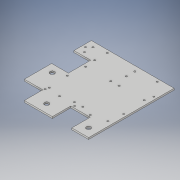
# Autodesk Inventor part: КВ33.044.002 - Дно платы
Saved by Autodesk Inventor 2019 (Build 230136000, 136)
## iProperties
Created: 2019-10-30
Part Number: КВ33.044.002 - Дно платы
Material: Типовые
Document SubType Name: Modeling
Designer: Петров Иван
Density: 1 g/cm^3
Appearance: По умолчанию
Mass: 56.5933 g
Surface Area: 408.613 cm^2
Volume: 56.5933 cm^3
Author: Петров Иван
Autodesk Inventor part; units mm, degrees
ref_plane "YZ Plane" through (0, 0, 0) normal (1, 0, 0) x (0, 1, 0)
ref_plane "XZ Plane" through (0, 0, 0) normal (0, 1, 0) x (-1, 0, 0)
ref_plane "XY Plane" through (0, 0, 0) normal (0, 0, 1) x (1, 0, 0)
sketch "Эскиз1" plane through (0, 0, 0) normal (0, 1, 0) x (-1, 0, 0)
  line L0 (-25, 35) -> (25, 35)
  line L1 (25, 35) -> (25, -35)
  line L2 (25, -35) -> (-25, -35)
  line L3 (-25, -35) -> (-25, 35)
  line L4 (-22.5, 32.5) -> (22.5, 32.5)
  line L5 (22.5, 31.5) -> (22.5, -31)
  line L6 (22.5, -32.5) -> (-22.5, -32.5)
  circle A0 centre (22.5, 32.5) radius 1.5
  circle A1 centre (22.5, -32.5) radius 1.5
  circle A2 centre (-22.5, -32.5) radius 1.5
  circle A3 centre (-22.5, 32.5) radius 1.5
  line L7 (-25, 35) -> (-23.7767, 33.2874) construction
  line L8 (-22.5, -31) -> (-22.5, 31)
  line L9 (23.7767, -33.2874) -> (25, -35) construction
  line L10 (25, -30.9585) -> (25, 35)
  line L11 (25, 35) -> (-25, 35)
  line L12 (25, 35) -> (25, -35)
  point P0 (0, 0)
  dimension "d6" = 3
  dimension "d0" = 50
  dimension "d2" = 45
  dimension "d4" = 3
  dimension "d5" = 3
  dimension "d7" = 3
  constraints: 26 end point, 4 coincident, 4 parallel, 4 point on circle, 3 centre point, 3 horizontal, 2 perpendicular, 2 point on line, 1 vertical alignment, 2 other
  measures "d0" distance of L1.end L2.end
  measures "d2" distance of L6.start L6.end
  measures "d4" diameter of A0
  measures "d5" diameter of A1
  measures "d7" diameter of A3
extrude "Выдавливание1" add sketch "Эскиз1" along normal blind 3 contours L0 L1 L2 L3 | L4 A0 L5 A1 L6 A2 L8 A3
sketch "Эскиз2" plane through (0, 3, 0) normal (0, 1, 0) x (1, 0, 0)
  line L0 (-25, -35) -> (25, -35) projected
  line L1 (-25, -35) -> (-28, -35)
  line L2 (-28, -35) -> (-28, 35)
  line L3 (-28, 35) -> (-25, 35)
  line L4 (-25, 35) -> (-25, -35)
  line L5 (-28, -35) -> (-58, -35)
  line L6 (-58, -35) -> (-58, 35)
  line L7 (-58, 35) -> (-28, 35)
  line L8 (-28, 35) -> (-28, -35)
  line L9 (-25, -35) -> (25, -35)
  line L10 (25, -35) -> (25, -38)
  line L11 (25, -38) -> (-25, -38)
  line L12 (-25, -38) -> (-25, -35)
  line L13 (-25, -38) -> (25, -38)
  line L14 (25, -38) -> (25, -68)
  line L15 (25, -68) -> (-25, -68)
  line L16 (-25, -68) -> (-25, -38)
  line L17 (-25, -68) -> (0, -68)
  line L18 (0, -53) -> (-25, -53)
  line L19 (-25, -53) -> (-25, -68)
  circle A0 centre (0, -53) radius 4
  line L20 (-58, 0) -> (-43, 0)
  circle A1 centre (-43, 0) radius 4
  point P0 (0, 0)
  dimension "d18" = 3
  dimension "d19" = 70
  dimension "d20" = 30
  dimension "d21" = 70
  dimension "d22" = 50
  dimension "d23" = 3
  dimension "d24" = 50
  dimension "d25" = 30
  dimension "d26" = 25
  dimension "d27" = 15
  dimension "d28" = 8
  dimension "d29" = 15
  dimension "d30" = 8
  constraints: 40 end point, 9 parallel, 6 horizontal, 4 perpendicular, 2 centre point, 2 coincident, 1 midpoint
  measures "d18" distance of L2.end L3.end
  measures "d19" distance of L1.end L2.end
  measures "d20" distance of L6.end L7.end
  measures "d21" distance of L5.end L6.end
  measures "d22" distance of L10.end L11.end
  measures "d23" distance of L9.end L10.end
  measures "d24" distance of L14.end L15.end
  measures "d25" distance of L13.end L14.end
  measures "d26" distance of L18.end L18.start
  measures "d27" distance of L18.start L17.end
  measures "d28" diameter of A0
  measures "d29" distance of L20.start L20.end
  measures "d30" diameter of A1
extrude "Выдавливание2" add sketch "Эскиз2" against normal blind 3
sketch "Эскиз3" plane through (0, 3, 0) normal (0, 1, 0) x (1, 0, 0)
  line L0 (-58, -35) -> (-25, -35) projected
  line L1 (-25, -35) -> (25, -35)
  line L2 (25, 35) -> (25, -68) projected
  line L3 (25, -35) -> (75, -35)
  line L4 (75, -35) -> (75, 35)
  line L5 (75, 35) -> (25, 35)
  line L6 (25, 35) -> (25, -35)
  point P0 (0, 0)
  dimension "d33" = 50
  constraints: 10 end point, 2 horizontal, 2 parallel, 1 perpendicular, 1 point on line
  measures "d33" distance of L5.end L4.end
extrude "Выдавливание3" add sketch "Эскиз3" against normal blind 3
move faces "Перенос1" translate (0, 0, -50) faces at (30.6667, 2, -35)
move faces "Перенос2" translate (15, 0, 0) faces at (75, 2, -5)
sketch "Эскиз6" plane through (0, 3, 0) normal (0, 1, 0) x (1, 0, 0)
  line L0 (-25, -35) -> (25, -35)
  line L1 (25, -35) -> (25, 35)
  line L2 (25, 35) -> (-25, 35)
  line L3 (-25, 35) -> (-25, -35)
  line L4 (-25, -35) -> (25, 35) construction
  line L5 (25, -35) -> (-25, 35) construction
  point P0 (0, 0)
  dimension "d46" = 50
  dimension "d47" = 70
  constraints: 12 end point, 2 midpoint, 2 parallel, 1 horizontal, 1 perpendicular
  measures "d46" distance of L2.end L1.end
  measures "d47" distance of L1.end L0.end
extrude "Выдавливание6" add sketch "Эскиз6" against normal blind 3
sketch "Эскиз7" plane through (0, 3, 0) normal (0, 1, 0) x (1, 0, 0)
  line L0 (-25, 41.6193) -> (25, 41.6193)
  line L1 (25, 41.6193) -> (25, -28.3807)
  line L2 (25, -28.3807) -> (-25, -28.3807)
  line L3 (-25, -28.3807) -> (-25, 41.6193)
  line L4 (-22.5, 39.1193) -> (22.5, 39.1193)
  line L5 (22.5, 38.1193) -> (22.5, -24.3807)
  line L6 (22.5, -25.8807) -> (-22.5, -25.8807)
  circle A0 centre (22.5, 39.1193) radius 1.5
  circle A1 centre (22.5, -25.8807) radius 1.5
  circle A2 centre (-22.5, -25.8807) radius 1.5
  circle A3 centre (-22.5, 39.1193) radius 1.5
  line L7 (-25, 41.6193) -> (-23.7767, 39.9067) construction
  line L8 (-22.5, -24.3807) -> (-22.5, 37.6193)
  line L9 (23.7767, -26.6681) -> (25, -28.3807) construction
  line L10 (25, -24.3391) -> (25, 41.6193)
  line L11 (25, 41.6193) -> (-25, 41.6193)
  line L12 (25, 41.6193) -> (25, -28.3807)
  point P0 (0, 0)
  point P1 (0, 6.6193)
  dimension "d54" = 3
  dimension "d50" = 50
  dimension "d51" = 45
  dimension "d52" = 3
  dimension "d53" = 3
  dimension "d55" = 3
  constraints: 26 end point, 4 coincident, 4 parallel, 4 point on circle, 3 centre point, 3 horizontal, 2 perpendicular, 2 point on line, 1 vertical alignment, 2 other
  measures "d50" distance of L1.end L2.end
  measures "d51" distance of L6.start L6.end
  measures "d52" diameter of A0
  measures "d53" diameter of A1
  measures "d55" diameter of A3
extrude "Выдавливание7" cut sketch "Эскиз7" against normal blind 3 contours A3 | A0 | A2 | A1
sketch "Эскиз8" plane through (0, 3, 0) normal (0, 1, 0) x (1, 0, 0)
  circle A0 centre (-46.0635, 75.8151) radius 1.5
  circle A1 centre (-46.0635, 60.8151) radius 1.5
  circle A2 centre (28.9365, 60.8151) radius 1.5
  circle A3 centre (28.9365, 75.8151) radius 1.5
  point P0 (0, 0)
  point P1 (-16.0911, 67.0392)
  dimension "d60" = 3
  dimension "d61" = 3
  dimension "d62" = 3
  dimension "d63" = 3
  dimension "d64" = 15
  dimension "d65" = 75
  dimension "d68" = 75
  constraints: 4 centre point
  measures "d60" diameter of A0
  measures "d61" diameter of A1
  measures "d62" diameter of A2
  measures "d63" diameter of A3
  measures "d64" distance of A2.centre A3.centre
  measures "d65" distance of A0.centre A3.centre
  measures "d68" distance of A2.centre A1.centre
extrude "Выдавливание8" cut sketch "Эскиз8" against normal blind 3
sketch "Эскиз9" plane through (0, 3, 0) normal (0, 1, 0) x (1, 0, 0)
  line L0 (-58, -35) -> (-58, 85) projected
  line L1 (-58, 13.7892) -> (-28, 13.7892)
  line L2 (-28, 13.7892) -> (-28, 53.7892)
  line L3 (-28, 53.7892) -> (-58, 53.7892)
  line L4 (-58, 53.7892) -> (-58, 13.7892)
  point P0 (0, 0)
  dimension "d69" = 30
  dimension "d70" = 40
  constraints: 8 end point, 2 parallel, 1 horizontal, 1 perpendicular, 1 point on line
  measures "d69" distance of L3.end L2.end
  measures "d70" distance of L2.end L1.end
extrude "Выдавливание9" cut sketch "Эскиз9" against normal blind 3
sketch "Эскиз10" plane through (0, 3, 0) normal (0, 1, 0) x (1, 0, 0)
  line L0 (90, 85) -> (90, -35) projected
  line L1 (90, -35) -> (60, -35)
  line L2 (60, -35) -> (60, -68)
  line L3 (60, -68) -> (90, -68)
  line L4 (90, -68) -> (90, -35)
  circle A0 centre (75, -53) radius 4
  point P0 (0, 0)
  dimension "d73" = 30
  dimension "d74" = 33
  dimension "d75" = 8
  dimension "d109" = 15
  dimension "d110" = 15
  constraints: 8 end point, 2 parallel, 1 centre point, 1 horizontal, 1 perpendicular
  measures "d73" distance of L3.end L2.end
  measures "d74" distance of L2.end L1.end
  measures "d75" diameter of A0
  measures "d109" distance from line of L3 A0.centre
  measures "d110" distance from line of L2 A0.centre
extrude "Выдавливание10" add sketch "Эскиз10" against normal blind 3
sketch "Эскиз11" plane through (0, 3, 0) normal (0, 1, 0) x (1, 0, 0)
  line L0 (-58, -35) -> (-25, -35) projected
  line L1 (60, -35) -> (25, -35) projected
  line L2 (-25, -35) -> (25, -35)
  line L3 (0, -35) -> (0, -30)
  circle A0 centre (0, -30) radius 1.5
  line L4 (-28, 13.7892) -> (-28, 53.7892) projected
  circle A1 centre (-25, 8.7892) radius 1.5
  line L5 (-58, 53.7892) -> (-58, 85) projected
  line L6 (-58, 69.3946) -> (-53, 69.3946)
  circle A2 centre (-53, 69.3946) radius 1.5
  line L7 (-28, 53.7892) -> (-58, 53.7892) projected
  line L8 (-28, 53.7892) -> (-24.4645, 57.3247)
  line L9 (-28, 53.7892) -> (-23, 53.7892) construction
  circle A3 centre (-24.4645, 57.3247) radius 1.5
  line L10 (-24.4645, 57.3247) -> (-24.4645, 85)
  line L11 (-58, 85) -> (90, 85) projected
  line L12 (-24.4645, 85) -> (-24.4645, 80)
  circle A4 centre (-24.4645, 80) radius 1.5
  line L13 (65, 85) -> (65, 80)
  circle A5 centre (65, 80) radius 1.5
  line L14 (90, -68) -> (90, 85) projected
  line L15 (90, 85) -> (90, -68) projected
  line L16 (90, 53.7892) -> (85, 53.7892)
  circle A6 centre (85, 53.7892) radius 1.5
  line L17 (60, -35) -> (90, -35)
  line L18 (90, 0) -> (85, 0)
  circle A7 centre (85, 0) radius 1.5
  line L19 (25, -35) -> (25, -68) projected
  line L20 (25, -35) -> (28.5355, -31.4645)
  line L21 (25, -35) -> (30, -35) construction
  circle A8 centre (28.5355, -31.4645) radius 1.5
  line L22 (60, -35) -> (56.4645, -31.4645)
  line L23 (60, -35) -> (65, -35) construction
  circle A9 centre (56.4645, -31.4645) radius 1.5
  line L24 (-24, -35) -> (-24, -32)
  circle A10 centre (-24, -32) radius 1.5
  line L25 (-28, 13.7892) -> (-58, 13.7892) projected
  line L26 (-58, 13.7892) -> (-58, -35) projected
  point P0 (0, 0)
  dimension "d78" = 5
  dimension "d79" = 3
  dimension "d81" = 3
  dimension "d82" = 5
  dimension "d83" = 3
  dimension "d84" = 5
  dimension "d85" = 45
  dimension "d86" = 3
  dimension "d87" = 5
  dimension "d88" = 3
  dimension "d89" = 5
  dimension "d90" = 3
  dimension "d91" = 25
  dimension "d92" = 5
  dimension "d93" = 3
  dimension "d94" = 5
  dimension "d95" = 3
  dimension "d96" = 5
  dimension "d97" = 45
  dimension "d98" = 3
  dimension "d99" = 5
  dimension "d100" = 135
  dimension "d101" = 3
  dimension "d102" = 3
  dimension "d103" = 3
  dimension "d106" = 5
  dimension "d107" = 3
  dimension "d108" = 34
  constraints: 32 end point, 11 centre point, 10 coincident, 7 point on line, 4 horizontal, 4 vertical, 3 equal length, 3 perpendicular, 2 midpoint, 1 collinear
  measures "d78" distance of L3.start L3.end
  measures "d79" diameter of A0
  measures "d81" diameter of A1
  measures "d82" distance of L6.start L6.end
  measures "d83" diameter of A2
  measures "d84" distance of L4.end L8.end
  measures "d85" angle of L9 L8
  measures "d86" diameter of A3
  measures "d87" distance of L10.end L12.end
  measures "d88" diameter of A4
  measures "d89" distance of L13.start L13.end
  measures "d90" diameter of A5
  measures "d91" distance between parallel lines of L14 L13
  measures "d92" distance of L16.start L16.end
  measures "d93" diameter of A6
  measures "d94" distance of L18.start L18.end
  measures "d95" diameter of A7
  measures "d96" distance of L1.end L20.end
  measures "d97" angle of L21 L20
  measures "d98" diameter of A8
  measures "d99" distance of L1.start L22.end
  measures "d100" angle of L23 L22
  measures "d101" diameter of A9
  measures "d102" distance of L24.start L24.end
  measures "d103" diameter of A10
  measures "d106" distance from line of L25 A1.centre
  measures "d107" distance from line of A1.centre L4
  measures "d108" distance between parallel lines of L26 L24
extrude "Выдавливание11" cut sketch "Эскиз11" against normal blind 10 contours A3 L10 L8 | L8 L10 A3 | A4 L10 | L10 A4 | A0 | A1 | A2 | A5 | A6 | A7 | A8 | A9 | A10
sketch "Эскиз12" plane through (0, 3, 0) normal (0, 1, 0) x (1, 0, 0)
  line L0 (34.4931, 42.1352) -> (84.4931, 42.1352)
  line L1 (84.4931, 42.1352) -> (84.4931, -27.8648)
  line L2 (84.4931, -27.8648) -> (34.4931, -27.8648)
  line L3 (34.4931, -27.8648) -> (34.4931, 42.1352)
  line L4 (36.9931, 39.6352) -> (81.9931, 39.6352)
  line L5 (81.9931, 38.6352) -> (81.9931, -23.8648)
  line L6 (81.9931, -25.3648) -> (36.9931, -25.3648)
  circle A0 centre (81.9931, 39.6352) radius 1.5
  circle A1 centre (81.9931, -25.3648) radius 1.5
  circle A2 centre (36.9931, -25.3648) radius 1.5
  circle A3 centre (36.9931, 39.6352) radius 1.5
  line L7 (34.4931, 42.1352) -> (35.7164, 40.4226) construction
  line L8 (36.9931, -23.8648) -> (36.9931, 38.1352)
  line L9 (83.2698, -26.1522) -> (84.4931, -27.8648) construction
  line L10 (84.4931, -23.8233) -> (84.4931, 42.1352)
  line L11 (84.4931, 42.1352) -> (34.4931, 42.1352)
  line L12 (84.4931, 42.1352) -> (84.4931, -27.8648)
  point P0 (0, 0)
  point P1 (59.4931, 0.5158)
  point P2 (59.4931, 7.1352)
  dimension "d115" = 3
  dimension "d111" = 50
  dimension "d112" = 45
  dimension "d113" = 3
  dimension "d114" = 3
  dimension "d116" = 3
  constraints: 26 end point, 4 coincident, 4 parallel, 4 point on circle, 3 centre point, 3 horizontal, 2 perpendicular, 2 point on line, 1 vertical alignment, 2 other
  measures "d111" distance of L1.end L2.end
  measures "d112" distance of L6.start L6.end
  measures "d113" diameter of A0
  measures "d114" diameter of A1
  measures "d116" diameter of A3
extrude "Выдавливание12" cut sketch "Эскиз12" against normal blind 10 contours A3 | A0 | A2 | A1
